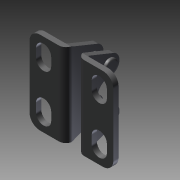
# Autodesk Inventor part: 205-S-WF
Saved by Autodesk Inventor 2011 SP1 (Build 150282100, 282)
## iProperties
Created: 2017-03-01
Part Number: 205-S-WF
Catalog Web Link: www.cadenas.de
Description: WF-SU-Winkelfuss
Vendor: DESTACO
Document SubType Name: Modeling
Designer: psAdmin
Manufacturer: DESTACO
Mass: 1.03269 g
Surface Area: 17.1279 cm^2
Volume: 1.03269 cm^3
Density: 1 g/cm^3
Category: PARTsolutions
Company: DESTACO
Title: 205-S-WF
Author: Cadenas PARTsolutions
Comments: Winkelfuss
PSOL_IDENT_0: {$CADENAS_DATA\23d-libs\destaco\destaco_gmbh\man_spann\horizontalspanner\standard\su_parts\winkelfus
PSOL_IDENT_1: s_su.prj},159 {VTYP=3D},{NB=205-S-WF},{LINA=205-S-WF},{NN=WF-SU},{DATE=20.09.2016 07:53:12},{GEOMDAT
PSOL_IDENT_2: E=20.03.2008 10:47:00},{VERSION=v1},{LINEID=20},{LINESUBID=-1},{WBVAR=}  {NB=205-S-WF},{LINA=205-S-W
PSOL_IDENT_3: F},{KT=DUMMY},{MODELL=205-S-WF},{HALTEKRAFT=250},{OEFFNUNG=90°},{GEWICHT=0.03},{ANDRUCKSPINDEL=20520
PSOL_IDENT_4: 8-M},{A=11.2},{A1=24.0},{A2=0.0},{A3=4.0},{A4=2.4},{A5=7.5},{B=16.0},{B1=23.5},{B3=4.3},{C=9.5},{C1=
PSOL_IDENT_5: 3.0},{C2=1.5},{F=4.2},{H=17.0},{L=69.5},{L1=21.5},{L2=16.5},{L3=0.0},{M=M4},{SIZE=1},{MOD=1.000},{VE
PSOL_IDENT_6: RS=1.000}
NN: WF-SU
NT: Winkelfuss
NB: 205-S-WF
NBSYN: $MODELL.
LINA: 205-S-WF
MODELL: 205-S-WF
HALTEKRAFT: 250
OEFFNUNG: 90°
GEWICHT: 0.03
ANDRUCKSPINDEL: 205208-M
A: 11.2
A1: 24.0
A2: 0.0
A3: 4.0
A4: 2.4
A5: 7.5
B: 16.0
B1: 23.5
B3: 4.3
C: 9.5
C1: 3.0
C2: 1.5
F: 4.2
H: 17.0
L: 69.5
L1: 21.5
L2: 16.5
L3: 0.0
M: M4
SIZE: 1
MOD: 1.000
VERS: 1.000
SUPPLIER: DESTACO
ARTICLENO: 205-S-WF
BOMINFO: 205-S-WF
CREATOR: CADENAS GmbH
Autodesk Inventor part; units mm, degrees
sketch "Skizze_1" plane through (0, 0, 0) normal (0, 0, 1) x (1, 0, 0)
  arc A0 (1.55, 2.1) -> (3.65, 0) centre (3.65, 2.1) ccw
  line L0 (3.65, 0) -> (12.05, 0)
  line L1 (12.05, 0) -> (12.05, 1.5)
  line L2 (12.05, 1.5) -> (3.65, 1.5)
  arc A1 (3.05, 2.1) -> (3.65, 1.5) centre (3.65, 2.1) ccw
  line L3 (3.05, 2.1) -> (3.05, 10.674)
  line L4 (3.05, 10.674) -> (1.55, 10.674)
  line L5 (1.55, 10.674) -> (1.55, 2.1)
  constraints: 12 end point, 4 point on circle, 2 centre point
extrude "Extrusion1" add sketch "Skizze_1" along normal blind 23.876
sketch "Skizze_2" plane through (0, 7.905, 0) normal (0, 1, 0) x (1, 0, 0)
  line L0 (-3.8374, -5.588) -> (3.8374, -5.588)
  line L1 (3.8374, -5.588) -> (3.8374, -6.993)
  arc A0 (3.3374, -7.493) -> (3.8374, -6.993) centre (3.3374, -6.993) ccw
  line L2 (3.3374, -7.493) -> (3.05, -7.493)
  line L3 (3.05, -7.493) -> (3.05, -7.1945)
  arc A1 (3.05, -7.1945) -> (2.65, -6.7945) centre (2.65, -7.1945) ccw
  line L4 (2.65, -6.7945) -> (-2.65, -6.7945)
  arc A2 (-2.65, -6.7945) -> (-3.05, -7.1945) centre (-2.65, -7.1945) ccw
  line L5 (-3.05, -7.1945) -> (-3.05, -7.493)
  line L6 (-3.05, -7.493) -> (-3.3374, -7.493)
  arc A3 (-3.8374, -6.993) -> (-3.3374, -7.493) centre (-3.3374, -6.993) ccw
  line L7 (-3.8374, -6.993) -> (-3.8374, -5.588)
  line L8 (-3.8374, -5.588) -> (3.8374, -5.588)
  constraints: 18 end point, 8 point on circle, 4 centre point
revolve "Revolution1" add sketch "Skizze_2" angle 360 about axis through (-3.8374, 7.905, 5.588) along (-1, 0, 0)
sketch "Skizze_3" plane through (0, 7.905, 0) normal (0, 1, 0) x (1, 0, 0)
  line L0 (-3.8374, -18.288) -> (3.8374, -18.288)
  line L1 (3.8374, -18.288) -> (3.8374, -19.693)
  arc A0 (3.3374, -20.193) -> (3.8374, -19.693) centre (3.3374, -19.693) ccw
  line L2 (3.3374, -20.193) -> (3.05, -20.193)
  line L3 (3.05, -20.193) -> (3.05, -19.8945)
  arc A1 (3.05, -19.8945) -> (2.65, -19.4945) centre (2.65, -19.8945) ccw
  line L4 (2.65, -19.4945) -> (-2.65, -19.4945)
  arc A2 (-2.65, -19.4945) -> (-3.05, -19.8945) centre (-2.65, -19.8945) ccw
  line L5 (-3.05, -19.8945) -> (-3.05, -20.193)
  line L6 (-3.05, -20.193) -> (-3.3374, -20.193)
  arc A3 (-3.8374, -19.693) -> (-3.3374, -20.193) centre (-3.3374, -19.693) ccw
  line L7 (-3.8374, -19.693) -> (-3.8374, -18.288)
  line L8 (-3.8374, -18.288) -> (3.8374, -18.288)
  constraints: 18 end point, 8 point on circle, 4 centre point
revolve "Revolution2" add sketch "Skizze_3" angle 360 about axis through (-3.8374, 7.905, 18.288) along (-1, 0, 0)
sketch "Skizze_4" plane through (0, 0, 0) normal (0, 0, 1) x (1, 0, 0)
  line L0 (-12.05, 1.5) -> (-12.05, 0)
  line L1 (-12.05, 0) -> (-3.65, 0)
  arc A0 (-3.65, 0) -> (-1.55, 2.1) centre (-3.65, 2.1) ccw
  line L2 (-1.55, 2.1) -> (-1.55, 10.674)
  line L3 (-1.55, 10.674) -> (-3.05, 10.674)
  line L4 (-3.05, 10.674) -> (-3.05, 2.1)
  arc A1 (-3.65, 1.5) -> (-3.05, 2.1) centre (-3.65, 2.1) ccw
  line L5 (-3.65, 1.5) -> (-12.05, 1.5)
  constraints: 12 end point, 4 point on circle, 2 centre point
extrude "Extrusion2" add sketch "Skizze_4" along normal blind 23.876
sketch "Skizze_5" plane through (0, 0, 0) normal (1, 0, 0) x (0, 1, 0)
  line L0 (-7, 30) -> (-7, -7)
  line L1 (-7, -7) -> (15, -7)
  line L2 (15, -7) -> (15, 30)
  line L3 (15, 30) -> (-7, 30)
  line L4 (1.5, 23.876) -> (0, 23.876)
  line L5 (0, 23.876) -> (0, 0)
  line L6 (0, 0) -> (1.5, 0)
  line L7 (1.5, 0) -> (9.029, 3.0378)
  arc A0 (9.029, 3.0378) -> (8, 8.338) centre (8, 5.588) ccw
  arc A1 (4.4, 11.938) -> (8, 8.338) centre (8, 11.938) ccw
  arc A2 (8, 15.538) -> (4.4, 11.938) centre (8, 11.938) ccw
  arc A3 (8, 15.538) -> (9.029, 20.8382) centre (8, 18.288) ccw
  line L8 (9.029, 20.8382) -> (1.5, 23.876)
  constraints: 18 end point, 8 point on circle, 4 centre point
extrude "Extrusion3" cut sketch "Skizze_5" along normal mid plane 50
sketch "Skizze_6" plane through (0, 0, 0) normal (0, 1, 0) x (-1, 0, 0)
  line L0 (31, 46) -> (-49, 46)
  line L1 (-49, 46) -> (-49, -17)
  line L2 (-49, -17) -> (31, -17)
  line L3 (31, -17) -> (31, 46)
  arc A0 (12.05, 20.876) -> (9.05, 23.876) centre (9.05, 20.876) ccw
  line L4 (9.05, 23.876) -> (-9.05, 23.876)
  arc A1 (-9.05, 23.876) -> (-12.05, 20.876) centre (-9.05, 20.876) ccw
  line L5 (-12.05, 20.876) -> (-12.05, 3)
  arc A2 (-12.05, 3) -> (-9.05, 0) centre (-9.05, 3) ccw
  line L6 (-9.05, 0) -> (9.05, 0)
  arc A3 (9.05, 0) -> (12.05, 3) centre (9.05, 3) ccw
  line L7 (12.05, 3) -> (12.05, 20.876)
  constraints: 16 end point, 8 point on circle, 4 centre point
extrude "Extrusion4" cut sketch "Skizze_6" along normal blind 5
sketch "Skizze_7" plane through (0, 0, 0) normal (0, 1, 0) x (-1, 0, 0)
  arc A0 (-5.827, 6.337) -> (-10.1958, 6.337) centre (-8.0114, 6.337) ccw
  line L0 (-10.1958, 6.337) -> (-10.1958, 3.937)
  arc A1 (-10.1958, 3.937) -> (-5.827, 3.937) centre (-8.0114, 3.937) ccw
  line L1 (-5.827, 3.937) -> (-5.827, 6.337)
  constraints: 4 end point, 4 point on circle, 2 centre point
extrude "Extrusion5" cut sketch "Skizze_7" along normal blind 1.5
sketch "Skizze_8" plane through (0, 0, 0) normal (0, 1, 0) x (-1, 0, 0)
  line L0 (-5.827, 17.539) -> (-5.827, 19.939)
  arc A0 (-5.827, 19.939) -> (-10.1958, 19.939) centre (-8.0114, 19.939) ccw
  line L1 (-10.1958, 19.939) -> (-10.1958, 17.539)
  arc A1 (-10.1958, 17.539) -> (-5.827, 17.539) centre (-8.0114, 17.539) ccw
  constraints: 4 end point, 4 point on circle, 2 centre point
extrude "Extrusion6" cut sketch "Skizze_8" along normal blind 5
sketch "Skizze_10" plane through (0, 0, 0) normal (0, 1, 0) x (-1, 0, 0)
  arc A0 (10.1958, 6.337) -> (5.827, 6.337) centre (8.0114, 6.337) ccw
  line L0 (5.827, 6.337) -> (5.827, 3.937)
  arc A1 (5.827, 3.937) -> (10.1958, 3.937) centre (8.0114, 3.937) ccw
  line L1 (10.1958, 3.937) -> (10.1958, 6.337)
  constraints: 4 end point, 4 point on circle, 2 centre point
extrude "Extrusion7" cut sketch "Skizze_10" along normal blind 5
sketch "Skizze_11" plane through (0, 0, 0) normal (0, 1, 0) x (-1, 0, 0)
  line L0 (10.1958, 17.539) -> (10.1958, 19.939)
  arc A0 (10.1958, 19.939) -> (5.827, 19.939) centre (8.0114, 19.939) ccw
  line L1 (5.827, 19.939) -> (5.827, 17.539)
  arc A1 (5.827, 17.539) -> (10.1958, 17.539) centre (8.0114, 17.539) ccw
  constraints: 4 end point, 4 point on circle, 2 centre point
extrude "Extrusion8" cut sketch "Skizze_11" along normal blind 3
ref_plane "WF1_XY" through (0, 7.905, 5.588) normal (1, 0, 0) x (0, 0, -1)
ref_plane "WF1_YZ" through (0, 7.905, 5.588) normal (0, 0, -1) x (0, 1, 0)
ref_plane "WF1_ZX" through (0, 7.905, 5.588) normal (0, 1, 0) x (1, 0, 0)
ref_plane "WF2_XY" through (0, 7.905, 18.288) normal (1, 0, 0) x (0, 0, -1)
ref_plane "WF2_YZ" through (0, 7.905, 18.288) normal (0, 0, -1) x (0, 1, 0)
ref_plane "WF2_ZX" through (0, 7.905, 18.288) normal (0, 1, 0) x (1, 0, 0)
body "Solid1"
